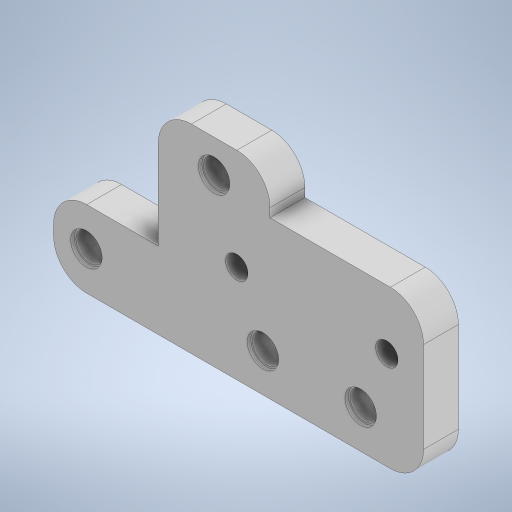
# Autodesk Inventor part: Hotend Mount
Saved by Autodesk Inventor 2023.1 (Build 271208000, 208)
## iProperties
Created: 2022-11-02
Part Number: Hotend Mount
Material: Generic
Document SubType Name: Modeling
Designer: nicol
Density: 1 g/cm^3
Appearance: Default
Author: nicol
Autodesk Inventor part; units mm, degrees
ref_plane "YZ Plane" through (0, 0, 0) normal (1, 0, 0) x (0, 1, 0)
ref_plane "XZ Plane" through (0, 0, 0) normal (0, 1, 0) x (-1, 0, 0)
ref_plane "XY Plane" through (0, 0, 0) normal (0, 0, 1) x (1, 0, 0)
sketch "Sketch1" plane through (0, 0, 0) normal (0, 0, 1) x (1, 0, 0)
  line L0 (0, 0) -> (44, 0)
  line L1 (44, 0) -> (44, 22.5)
  line L2 (44, 22.5) -> (0, 22.5)
  line L3 (0, 22.5) -> (0, 0)
  line L4 (29, 5.5) -> (44, 5.5) construction
  line L5 (15, 5.5) -> (0, 5.5) construction
  line L6 (32.75, 14) -> (44, 14) construction
  line L7 (11.25, 14) -> (0, 14) construction
  line L8 (0, 11) -> (-15, 11)
  line L9 (-15, 11) -> (-15, 0)
  line L10 (-15, 0) -> (0, 0)
  line L11 (0, 0) -> (0, 11)
  line L12 (0, 22.5) -> (16, 22.5)
  line L13 (16, 22.5) -> (16, 28.5)
  line L14 (16, 28.5) -> (0, 28.5)
  line L15 (0, 28.5) -> (0, 22.5)
  point P0 (8, 23.8)
  point P1 (-10.3, 5.5)
  point P2 (-15, 5.5)
  point P3 (8, 28.5)
  dimension "d0" = 14
  dimension "d1" = 21.5
  dimension "d2" = 18.3
  dimension "d3" = 18.3
  dimension "d5" = 7
  dimension "d6" = 44
  dimension "d10" = 15
  dimension "d11" = 8
  dimension "d13" = 22.5
  dimension "d28" = 4.7
  dimension "d43" = 5.5
  dimension "d44" = 8.5
  dimension "d45" = 8.5
  constraints: 32 end point, 6 parallel, 6 point on line, 5 perpendicular, 4 horizontal, 4 horizontal alignment, 3 collinear, 2 midpoint, 1 vertical alignment
  measures "d0" distance of L5.start L4.start
  measures "d1" distance of L7.start L6.start
  measures "d2" horizontal distance of point (-10.3, 5.5) point (8, 23.8)
  measures "d3" horizontal distance of point (-10.3, 5.5) point (8, 23.8)
  measures "d5" horizontal distance of point (8, 23.8) L5.start
  measures "d6" distance of L0.start L0.end
  measures "d10" distance of L8.start L8.end
  measures "d11" distance from line of L3 point (8, 23.8)
  measures "d13" distance of L0.end L1.end
  measures "d28" distance from line of L14 point (8, 23.8)
  measures "d43" distance from line of L0 L5.start
  measures "d44" distance from line of L5 L7.start
  measures "d45" distance from line of L12 L7.start
extrude "Extrusion1" add sketch "Sketch1" against normal blind 5
hole "Hole1" at (15, 5.5, 0) at (29, 5.5, 0) at (8, 23.8, 0) at (-10.3, 5.5, 0) direction (0, 0, -1) diameter 4 end through all counterbore diameter 4.5 counterbore depth 0.5
sketch "Sketch2" plane through (0, 0, 0) normal (0, 0, 1) x (1, 0, 0)
  line L0 (38, 26.3081) -> (49.0183, 26.3081)
  line L1 (49.0183, 26.3081) -> (49.0183, -7.071)
  line L2 (49.0183, -7.071) -> (38, -7.071)
  line L3 (38, -7.071) -> (38, 26.3081)
  line L4 (44, 0) -> (44, 22.5) projected
  point P0 (0, 0)
  dimension "d29" = 6
  constraints: 8 end point, 2 parallel, 1 horizontal, 1 perpendicular
  measures "d29" distance between parallel lines of L3 L4
extrude "Extrusion2" cut sketch "Sketch2" against normal through all
hole "Hole2" at (11.25, 14, 0) at (32.75, 14, 0) direction (0, 0, -1) diameter 3.2 end through all
fillet "Fillet1" radius 4.75 6 edges at (38, 22.5, -2.5) (16, 28.5, -2.5) (0, 28.5, -2.5) (-15, 11, -2.5) (-15, 0, -2.5) (38, 0, -2.5)
equation "\"d45\" = d44"
body "Solid1"
